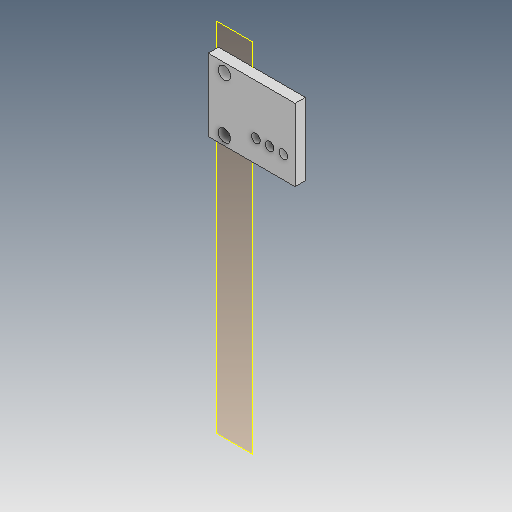
# Autodesk Inventor part: Limit switch mount top
Saved by Autodesk Inventor 2020 (Build 240168000, 168)
## iProperties
Created: 2019-11-21
Part Number: Limit switch mount top
Material: Generic
Document SubType Name: Modeling
Designer: ball
Density: 1 g/cm^3
Appearance: Default
Author: ball
Autodesk Inventor part; units mm, degrees
ref_plane "YZ Plane" through (0, 0, 0) normal (1, 0, 0) x (0, 1, 0)
ref_plane "XZ Plane" through (0, 0, 0) normal (0, 1, 0) x (-1, 0, 0)
ref_plane "XY Plane" through (0, 0, 0) normal (0, 0, 1) x (1, 0, 0)
ref_plane "Work Plane1" through (0, 0, 0) normal (0, 0, 1) x (1, 0, 0)
sketch "Sketch1" plane through (0, 0, 0) normal (0, 0, 1) x (1, 0, 0)
  circle A0 centre (4.5, -4) radius 1.45 construction
  circle A1 centre (4.5, -9) radius 1.45 construction
  circle A2 centre (4.5, -14) radius 1.45 construction
  circle A3 centre (4.5, -19) radius 1.45 construction
  circle A4 centre (4.5, -24) radius 1.45 construction
  circle A5 centre (4.5, -29) radius 1.45 construction
  circle A6 centre (4.5, -34) radius 1.45 construction
  circle A7 centre (4.5, -39) radius 1.45 construction
  line L0 (0, -90) -> (0, 0) construction
  line L1 (0, 0) -> (9, 0) construction
  line L2 (9, 0) -> (9, -90) construction
  line L3 (9, 0) -> (9, -90) construction
  line L4 (0, -21.5) -> (24.0956, -21.5)
  line L5 (24.0956, -21.5) -> (24.0956, -1.5)
  line L6 (24.0956, -1.5) -> (0, -1.5)
  line L7 (0, -1.5) -> (0, -21.5)
  circle A8 centre (4.5, -4) radius 1.7
  circle A9 centre (4.5, -19) radius 1.7
  circle A10 centre (17.037, -24.8666) radius 1.1938 construction
  circle A11 centre (17.037, -15.3416) radius 1.1938 construction
  circle A12 centre (17.037, -24.8666) radius 1.1938
  circle A13 centre (17.037, -15.3416) radius 1.1938
  circle A14 centre (20.847, -24.8666) radius 1.1938
  circle A15 centre (20.847, -15.3416) radius 1.1938
  circle A16 centre (13.227, -24.8666) radius 1.1938
  circle A17 centre (13.227, -15.3416) radius 1.1938
  circle A18 centre (17.037, -24.8666) radius 1.1938
  circle A19 centre (17.037, -15.3416) radius 1.1938
  dimension "d1" = 3.4
  dimension "d2" = 3.4
  dimension "d3" = 2.5
  dimension "d4" = 2.5
  dimension "d14" = 3.81
  dimension "d17" = 3.81
  constraints: 10 centre point, 8 end point, 4 coincident, 3 horizontal, 2 concentric, 2 parallel, 1 perpendicular, 1 point on line, 12 other
  measures "d1" diameter of A8
  measures "d2" diameter of A9
  measures "d3" distance from line of L4 A3.centre
  measures "d4" distance from line of A0.centre L6
  measures "d14" distance of A12.centre A14.centre
  measures "d17" distance of A12.centre A16.centre
ref_plane "Work Plane2" through (14.1732, -6.9151, 2.8702) normal (0, 0, -1) x (0, 1, 0)
extrude "Extrusion1" add sketch "Sketch1" along normal up to surface (2.8702 mm away) contours L7 L6 L5 L4
equation "\"d4\" = d3"
body "Solid1"
